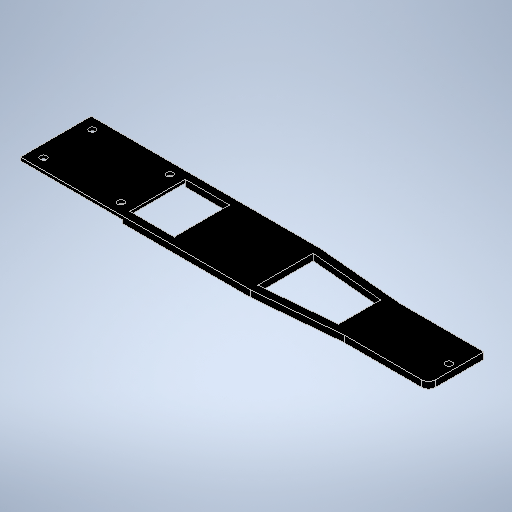
# Autodesk Inventor part: nakladkapart2
Saved by Autodesk Inventor 2025.3 (Build 293356000, 356)
## iProperties
Created: 2026-04-12
Part Number: nakladkapart2
Material: PCTG 20%
Document SubType Name: Modeling
Designer: ksawe
Density: 1.541 g/cm^3
Appearance: Anodized - Black
Author: ksawe
Autodesk Inventor part; units mm, degrees
ref_plane "YZ Plane" through (0, 0, 0) normal (1, 0, 0) x (0, 1, 0)
ref_plane "XZ Plane" through (0, 0, 0) normal (0, 1, 0) x (-1, 0, 0)
ref_plane "XY Plane" through (0, 0, 0) normal (0, 0, 1) x (1, 0, 0)
sketch "Sketch1" plane through (0, 0, 0) normal (0, 1, 0) x (-1, 0, 0)
  line L0 (-119.8086, 12.5082) -> (-80.837, 16)
  line L1 (-80.837, 16) -> (0, 16)
  line L2 (-120, 0) -> (120, 0) construction
  line L3 (-120, -12.4911) -> (-80.837, -16)
  line L4 (-80.837, -16) -> (0, -16)
  line L5 (0, 16) -> (0, -16) construction
  line L6 (80.837, 16) -> (0, 16)
  line L7 (119.8086, 12.5082) -> (80.837, 16)
  line L8 (120, -12.4911) -> (80.837, -16)
  line L9 (80.837, -16) -> (0, -16)
  line L10 (-80.837, -12.486) -> (-114.3086, -9.487)
  line L11 (-80.837, 12.486) -> (-114.3086, 9.487)
  line L12 (-114.3086, 9.487) -> (-114.3086, -9.487)
  line L13 (-80.837, 12.486) -> (-80.837, -12.486)
  line L14 (-23, 12.5) -> (-43, 12.5)
  line L15 (-43, 12.5) -> (-43, -12.5)
  line L16 (-43, -12.5) -> (-23, -12.5)
  line L17 (-23, -12.5) -> (-23, 12.5)
  line L18 (80.837, -12.486) -> (114.3086, -9.487)
  line L19 (80.837, 12.486) -> (114.3086, 9.487)
  line L20 (114.3086, 9.487) -> (114.3086, -9.487)
  line L21 (80.837, 12.486) -> (80.837, -12.486)
  line L22 (23, 12.5) -> (43, 12.5)
  line L23 (43, 12.5) -> (43, -12.5)
  line L24 (43, -12.5) -> (23, -12.5)
  line L25 (23, -12.5) -> (23, 12.5)
  circle A0 centre (-17.5, -11) radius 1.5
  circle A1 centre (17.5, -11) radius 1.5
  circle A2 centre (-17.5, 11) radius 1.5
  circle A3 centre (17.5, 11) radius 1.5
  line L26 (-119.8086, 12.5082) -> (-158, 12.5082)
  line L27 (-158, 12.5082) -> (-158, -12.4911)
  line L28 (-120, -12.4911) -> (-158, -12.4911)
  circle A4 centre (-154.68, 0) radius 1.5
  line L29 (119.8086, 12.5082) -> (158, 12.5082)
  line L30 (158, 12.5082) -> (158, -12.4911)
  line L31 (120, -12.4911) -> (158, -12.4911)
  circle A5 centre (154.68, 0) radius 1.5
  point P0 (0, 0)
  point P1 (0, 0)
  point P2 (0, 0)
  point P3 (-114.3086, 0)
  point P4 (-33, 12.5)
  dimension "d0" = 25
  dimension "d2" = 80.837
  dimension "d6" = 3.5
  dimension "d9" = 3.5
  dimension "d10" = 3.5
  dimension "d11" = 20
  dimension "d13" = 3
  dimension "d14" = 5
  dimension "d15" = 5.5
  dimension "d17" = 38
  dimension "d18" = 39.163
  dimension "d19" = 5.5
  dimension "d23" = 3
  dimension "d24" = 3.32
  dimension "d30" = 32
  dimension "d33" = 23
  dimension "d34" = 3.5089
  constraints: 64 end point, 22 symmetric about line, 6 centre point, 5 horizontal, 4 midpoint, 4 parallel, 3 coincident, 3 vertical, 2 perpendicular, 2 vertical alignment, 1 horizontal alignment, 4 other
  measures "d0" distance of L0.start L3.start
  measures "d2" distance of L0.end L1.end
  measures "d6" distance between parallel lines of L3 L10
  measures "d9" distance from line of L1 point (-33, 12.5)
  measures "d10" distance between parallel lines of L4 L16
  measures "d11" distance of L14.start L14.end
  measures "d13" diameter of A0
  measures "d14" distance from line of L4 A0.centre
  measures "d15" distance from line of L17 A0.centre
  measures "d17" distance of L3.start L27.end
  measures "d18" distance of L3.start L10.start
  measures "d19" horizontal distance of L0.start L11.end
  measures "d23" diameter of A4
  measures "d24" distance from line of L27 A4.centre
  measures "d30" distance between parallel lines of L1 L4
  measures "d33" distance from line of L17 point (0, 0)
  measures "d34" vertical distance of L3.start L3.end
extrude "Extrusion1" add sketch "Sketch1" along normal mid plane 3
fillet "Fillet1" radius 3 2 edges at (-158, 0, 12.5082) (158, 0, 12.5082)
sketch "Sketch3" plane through (-80.837, 1.5, 16) normal (0, 0, 1) x (1, 0, 0)
  line L0 (0, 0) -> (161.674, 0) projected
  line L1 (161.674, -3) -> (0, -3) projected
  line L2 (57.837, -3) -> (57.837, 0) projected
  line L3 (103.837, -3) -> (103.837, 0) projected
  line L4 (57.837, -3) -> (57.837, 0) projected
  line L5 (57.837, -1.5) -> (103.837, -1.5)
  line L6 (238.837, -3) -> (238.837, 0) projected
  line L7 (200.6456, 0) -> (235.837, 0) projected
  line L8 (235.837, 0) -> (238.837, 0) projected
  line L9 (238.837, -3) -> (235.837, -3) projected
  line L10 (235.837, -3) -> (200.6456, -3) projected
  line L11 (200.6456, -3) -> (161.674, -3) projected
  line L12 (161.674, 0) -> (200.6456, 0) projected
  line L13 (-38.9716, 0) -> (0, 0) projected
  line L14 (0, -3) -> (-38.9716, -3) projected
  line L15 (-74.163, 0) -> (-38.9716, 0) projected
  line L16 (-38.9716, -3) -> (-74.163, -3) projected
  line L17 (-77.163, 0) -> (-77.163, -3) projected
  line L18 (-74.163, -3) -> (-77.163, -3) projected
  line L19 (-77.163, 0) -> (-74.163, 0) projected
  point P0 (80.837, -1.5)
  constraints: 2 end point, 2 midpoint
extrude "Extrusion3" cut sketch "Sketch3" against normal through all contours L0 L2 L1 L14 L16 L18 L17 L19 L15 L13 | L5 L3 L1 L2
body "Solid1"
